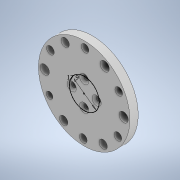
# Autodesk Inventor part: omniwheel_mount
Saved by Autodesk Inventor 2020 (Build 240168000, 168)
## iProperties
Created: 2020-01-03
Part Number: omniwheel_mount
Material: Generic
Document SubType Name: Modeling
Designer: my
Density: 1 g/cm^3
Appearance: Default
Author: my
Autodesk Inventor part; units mm, degrees
ref_plane "YZ Plane" through (0, 0, 0) normal (1, 0, 0) x (0, 1, 0)
ref_plane "XZ Plane" through (0, 0, 0) normal (0, 1, 0) x (-1, 0, 0)
ref_plane "XY Plane" through (0, 0, 0) normal (0, 0, 1) x (1, 0, 0)
sketch "Sketch1" plane through (0, 0, 0) normal (0, 0, 1) x (1, 0, 0)
  circle A0 centre (0, 0) radius 17.5
  dimension "d0" = 35
  constraints: 1 centre point, 1 coincident
  measures "d0" diameter of A0
extrude "Extrusion1" add sketch "Sketch1" along normal blind 2
sketch "Sketch2" plane through (0, 0, 2) normal (0, 0, 1) x (1, 0, 0)
  circle A0 centre (0, 0) radius 27.5
  dimension "d3" = 55
  constraints: 1 centre point, 1 coincident
  measures "d3" diameter of A0
extrude "Extrusion2" add sketch "Sketch2" along normal blind 5
fillet "Fillet1" radius 5 1 edges at (-17.5, 0, 2)
sketch "Sketch3" plane through (0, 0, 0) normal (0, 0, -1) x (-1, 0, 0)
  circle A0 centre (-12.3215, 20.3038) radius 2.8 projected
  circle A1 centre (-0.5188, 23.7443) radius 2.3 projected
  circle A2 centre (11.4228, 20.8226) radius 2.5 projected
  circle A3 centre (20.3038, 12.3215) radius 2.3 projected
  circle A4 centre (23.7443, 0.5188) radius 2.8 projected
  circle A5 centre (20.8226, -11.4228) radius 2 projected
  circle A6 centre (12.3215, -20.3038) radius 2.5 projected
  circle A7 centre (0.5188, -23.7443) radius 2.3 projected
  circle A8 centre (-11.4228, -20.8226) radius 2.5 projected
  circle A9 centre (-20.3038, -12.3215) radius 2.3 projected
  circle A10 centre (-23.7443, -0.5188) radius 2.8 projected
  circle A11 centre (-20.8226, 11.4228) radius 2.3 projected
extrude "Extrusion3" cut sketch "Sketch3" against normal blind 10
sketch "Sketch4" plane through (0, 0, 7) normal (0, 0, 1) x (1, 0, 0)
  circle A0 centre (0, 0) radius 8.95
  dimension "d9" = 17.9
  constraints: 1 centre point, 1 coincident
  measures "d9" diameter of A0
sketch "Sketch5" plane through (0, 0, 7) normal (0, 0, 1) x (1, 0, 0)
  circle A0 centre (0, 0) radius 7.5
  point P0 (7.5, 0)
  point P1 (0, 7.5)
  point P2 (-7.5, 0)
  point P3 (0, -7.5)
  dimension "d12" = 15
  constraints: 4 point on circle, 1 centre point, 1 coincident
  measures "d12" diameter of A0
hole "Hole2" at (7.5, 0, 7) at (0, 7.5, 7) at (-7.5, 0, 7) at (0, -7.5, 7) direction (0, 0, -1) diameter 2.9 depth 20 countersink diameter 5.5 countersink angle 90 clearance for "Countersunk Flat Head Screw ISO 2009/7046" size "M2.5" standard "ISO"
body "Solid1"
